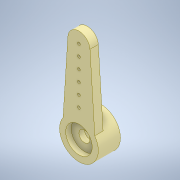
# Autodesk Inventor part: Arm 1
Saved by Autodesk Inventor 2021 (Build 250183000, 183)
## iProperties
Created: 2016-01-04
Part Number: Arm 1
Material: Нейлон 6/6
Document SubType Name: Modeling
Designer: Evgeny
Density: 1.13 g/cm^3
Appearance: Нейлон 6
Author: Evgeny
Autodesk Inventor part; units mm, degrees
ref_plane "YZ Plane" through (0, 0, 0) normal (1, 0, 0) x (0, 1, 0)
ref_plane "XZ Plane" through (0, 0, 0) normal (0, 1, 0) x (-1, 0, 0)
ref_plane "XY Plane" through (0, 0, 0) normal (0, 0, 1) x (1, 0, 0)
sketch "Эскиз1" plane through (0, 0, 0) normal (0, 1, 0) x (-1, 0, 0)
  circle A0 centre (0, 0) radius 1
  circle A1 centre (0, 0) radius 3.5
  arc A2 (1.9956, 15.1325) -> (-1.9956, 15.1325) centre (0, 15) ccw
  line L0 (1.9956, 15.1325) -> (2.8667, 2.008)
  line L1 (-1.9956, 15.1325) -> (-2.8667, 2.008)
  circle A3 centre (0, 15) radius 0.25
  circle A4 centre (0, 13) radius 0.25
  circle A5 centre (0, 11) radius 0.25
  circle A6 centre (0, 9) radius 0.25
  circle A7 centre (0, 7) radius 0.25
  circle A8 centre (0, 5) radius 0.25
  line L2 (2.8667, 2.008) -> (3, 0) construction
  line L3 (-2.8667, 2.008) -> (-3, 0) construction
  dimension "d0" = 7
  dimension "d1" = 2
  dimension "d2" = 3
  dimension "d3" = 3
  dimension "d4" = 15
  dimension "d5" = 2
  dimension "d6" = 0.5
  dimension "d7" = 0.5
  dimension "d8" = 0.5
  dimension "d9" = 0.5
  dimension "d10" = 0.5
  dimension "d11" = 0.5
  dimension "d13" = 2
  dimension "d14" = 2
  dimension "d15" = 2
  dimension "d16" = 2
  dimension "d17" = 2
  constraints: 9 centre point, 8 end point, 5 vertical alignment, 4 point on circle, 4 tangent, 3 coincident, 2 horizontal alignment
  measures "d0" diameter of A1
  measures "d1" diameter of A0
  measures "d2" distance of L2.end point (0, 0)
  measures "d3" distance of L3.end point (0, 0)
  measures "d4" distance of A2.centre point (0, 0)
  measures "d5" radius of A2
  measures "d6" diameter of A3
  measures "d7" diameter of A4
  measures "d8" diameter of A5
  measures "d9" diameter of A6
  measures "d10" diameter of A7
  measures "d11" diameter of A8
  measures "d13" distance of A4.centre A2.centre
  measures "d14" distance of A5.centre A4.centre
  measures "d15" distance of A6.centre A5.centre
  measures "d16" distance of A7.centre A6.centre
  measures "d17" distance of A8.centre A7.centre
extrude "Выдавливание1" add sketch "Эскиз1" along normal blind 1.5
sketch "Эскиз2" plane through (0, 1.5, 0) normal (0, 1, 0) x (1, 0, 0)
  arc A0 (2.8667, -2.008) -> (-2.8667, -2.008) centre (0, 0) ccw projected
  circle A1 centre (0, 0) radius 1 projected
  circle A2 centre (0, 0) radius 3.5
  constraints: 1 centre point, 1 coincident, 1 concentric
extrude "Выдавливание2" add sketch "Эскиз2" along normal blind 2.5
sketch "Эскиз3" plane through (0, 4, 0) normal (0, 1, 0) x (1, 0, 0)
  circle A0 centre (0, 0) radius 1 projected
  circle A1 centre (0, 0) radius 2.25
  dimension "d23" = 4.5
  constraints: 1 centre point, 1 coincident
  measures "d23" diameter of A1
extrude "Выдавливание3" cut sketch "Эскиз3" against normal blind 2
sketch "Эскиз4" plane through (0, 0, 0) normal (0, -1, 0) x (1, 0, 0)
  circle A0 centre (0, 0) radius 2.4
  dimension "d29" = 4.8
  constraints: 1 centre point, 1 coincident
  measures "d29" diameter of A0
extrude "Выдавливание4" cut sketch "Эскиз4" against normal blind 1
equation "\"d7\" = d6"
equation "\"d8\" = d6"
equation "\"d9\" = d6"
equation "\"d10\" = d6"
equation "\"d11\" = d6"
